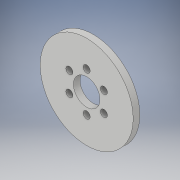
# Autodesk Inventor part: AZUSASprocketSmall
Saved by Autodesk Inventor 2019 (Build 230136000, 136)
## iProperties
Created: 2020-02-11
Part Number: AZUSASprocketSmall
Material: Generic
Document SubType Name: Modeling
Designer: rittmasm
Density: 1 g/cm^3
Appearance: Default
Author: rittmasm
Autodesk Inventor part; units mm, degrees
ref_plane "YZ Plane" through (0, 0, 0) normal (1, 0, 0) x (0, 1, 0)
ref_plane "XZ Plane" through (0, 0, 0) normal (0, 1, 0) x (-1, 0, 0)
ref_plane "XY Plane" through (0, 0, 0) normal (0, 0, 1) x (1, 0, 0)
sketch "Sketch1" plane through (0, 0, 0) normal (0, 0, 1) x (1, 0, 0)
  circle A0 centre (0, 0) radius 12.7
  circle A1 centre (0, 0) radius 44.45
  dimension "d0" = 25.4
  dimension "d1" = 88.9
  constraints: 2 centre point, 2 coincident
  measures "d0" diameter of A0
  measures "d1" diameter of A1
extrude "Extrusion1" add sketch "Sketch1" along normal blind 6.35
sketch "Sketch2" plane through (0, 0, 0) normal (0, 0, -1) x (-1, 0, 0)
  circle A0 centre (0, 0) radius 19.05
  circle A1 centre (0, -19.05) radius 3.3782
  circle A2 centre (16.4978, -9.525) radius 3.3782
  circle A3 centre (16.4978, 9.525) radius 3.3782
  circle A4 centre (0, 19.05) radius 3.3782
  circle A5 centre (-16.4978, 9.525) radius 3.3782
  circle A6 centre (-16.4978, -9.525) radius 3.3782
  dimension "d4" = 38.1
  dimension "d5" = 6.7564
  dimension "d8" = 360
  constraints: 6 centre point, 1 coincident, 1 vertical alignment, 15 other
  measures "d5" diameter of A1
extrude "Extrusion2" cut sketch "Sketch2" against normal blind 6.35 contours A3 A0 | A0 A3 | A2 A0 | A0 A2 | A4 A0 | A0 A4 | A1 A0 | A0 A1 | A5 A0 | A0 A5 | A6 A0 | A0 A6
body "Solid1"
